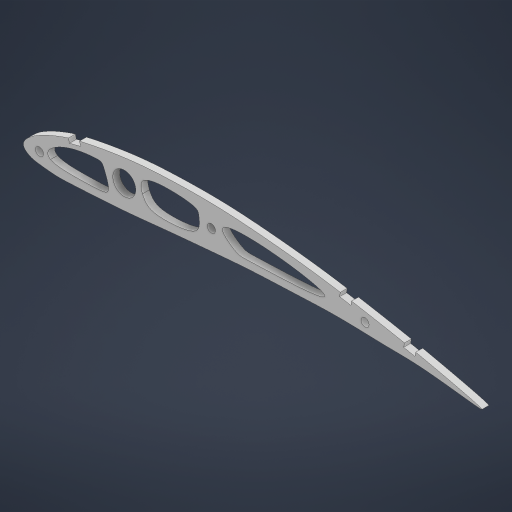
# Autodesk Inventor part: Żebro default
Saved by Autodesk Inventor 2023.2 (Build 272271000, 271)
## iProperties
Created: 2022-12-26
Part Number: Żebro default
Material: Generic
Document SubType Name: Modeling
Designer: Maciej
Density: 1 g/cm^3
Appearance: Default
Author: Maciej
Autodesk Inventor part; units mm, degrees
ref_plane "YZ Plane" through (0, 0, 0) normal (1, 0, 0) x (0, 1, 0)
ref_plane "XZ Plane" through (0, 0, 0) normal (0, 1, 0) x (-1, 0, 0)
ref_plane "XY Plane" through (0, 0, 0) normal (0, 0, 1) x (1, 0, 0)
sketch "Sketch1" plane through (0, 0, 0) normal (0, 0, 1) x (1, 0, 0)
  circle A0 centre (44, 7) radius 5
  spline S0 degree 5 poles (199.9996, -0.38) (200.0106, -0.3312) (199.8804, -0.2049) (199.2285, 0.0711) (197.4897, 0.603) (194.1404, 1.4843) (189.9902, 2.5038) (185.4529, 3.5751) (180.917, 4.6174) (176.6859, 5.5683) (172.905, 6.399) (169.5797, 7.1105) (166.6212, 7.7241) (163.8815, 8.2732) (161.1948, 8.7949) (158.4128, 9.3222) (155.4505, 9.8742) (152.2916, 10.4547) (148.9653, 11.0574) (145.5311, 11.6693) (142.0603, 12.2741) (138.6195, 12.856) (135.2509, 13.4043) (131.9642, 13.9143) (128.7482, 14.3862) (125.5772, 14.8234) (122.4201, 15.231) (119.2476, 15.6147) (116.0409, 15.9792) (112.7977, 16.3273) (109.526, 16.6598) (106.2399, 16.9761) (102.9553, 17.2744) (99.6851, 17.5515) (96.4347, 17.8034) (93.1983, 18.0254) (89.9631, 18.2128) (86.7143, 18.361) (83.4389, 18.467) (80.1306, 18.5292) (76.7936, 18.5484) (73.4478, 18.5285) (70.121, 18.4747) (66.842, 18.3921) (63.6325, 18.2845) (60.4998, 18.1522) (57.4298, 17.991) (54.3776, 17.7904) (51.2803, 17.5356) (48.0737, 17.2117) (44.708, 16.8059) (41.1643, 16.3117) (37.4684, 15.7314) (33.7125, 15.0801) (30.0381, 14.3833) (26.6017, 13.6712) (23.5476, 12.9739) (20.9752, 12.316) (18.9135, 11.7124) (17.2802, 11.1621) (15.8986, 10.6463) (14.5706, 10.1314) (13.1408, 9.567) (11.5443, 8.8974) (9.8001, 8.0944) (8.0206, 7.1907) (6.4035, 6.3015) (5.1063, 5.5301) (4.1412, 4.8917) (3.2339, 4.2107) (2.0734, 3.2532) (0.7635, 1.9494) (-0.1408, 0.4578) (-0.11, -0.9841) (0.869, -2.1755) (2.225, -3.0309) (3.3947, -3.5548) (4.3703, -3.8516) (5.5295, -4.0649) (7.0665, -4.2813) (8.8743, -4.5078) (10.739, -4.7168) (12.4766, -4.8786) (14.0301, -4.9827) (15.4348, -5.0277) (16.824, -5.0185) (18.3985, -4.9615) (20.3559, -4.8641) (22.8188, -4.7325) (25.7852, -4.5706) (29.1702, -4.381) (32.834, -4.1653) (36.6154, -3.9248) (40.3617, -3.661) (43.9625, -3.3764) (47.3772, -3.075) (50.6165, -2.7615) (53.7267, -2.4408) (56.7726, -2.1177) (59.8215, -1.7961) (62.9264, -1.4784) (66.1089, -1.1652) (69.3663, -0.8558) (72.679, -0.5487) (76.0189, -0.2431) (79.3565, 0.0615) (82.6686, 0.3634) (85.9473, 0.6587) (89.1972, 0.9419) (92.4304, 1.2068) (95.6623, 1.4479) (98.9069, 1.6618) (102.1727, 1.8475) (105.4574, 2.0086) (108.7492, 2.1521) (112.0324, 2.2861) (115.292, 2.4185) (118.5181, 2.5543) (121.7099, 2.6948) (124.8823, 2.8347) (128.0632, 2.9627) (131.2839, 3.0653) (134.5721, 3.1297) (137.9424, 3.1463) (141.3901, 3.1121) (144.8796, 3.0338) (148.3468, 2.9283) (151.7203, 2.8162) (154.9369, 2.7175) (157.9613, 2.6462) (160.8018, 2.6058) (163.5319, 2.5834) (166.2946, 2.5476) (169.2559, 2.4601) (172.5682, 2.2839) (176.329, 1.9925) (180.5433, 1.5794) (185.08, 1.0675) (189.6443, 0.5164) (193.8498, 0.0059) (197.2799, -0.3763) (199.0986, -0.515) (199.8149, -0.4977) (199.9887, -0.4288) (199.9996, -0.38) knots 0 0 0 0 0 0 0.007143 0.014286 0.021429 0.028571 0.035714 0.042857 0.05 0.057143 0.064286 0.071429 0.078571 0.085714 0.092857 0.1 0.107143 0.114286 0.121429 0.128571 0.135714 0.142857 0.15 0.157143 0.164286 0.171429 0.178571 0.185714 0.192857 0.2 0.207143 0.214286 0.221429 0.228571 0.235714 0.242857 0.25 0.257143 0.264286 0.271429 0.278571 0.285714 0.292857 0.3 0.307143 0.314286 0.321429 0.328571 0.335714 0.342857 0.35 0.357143 0.364286 0.371429 0.378571 0.385714 0.392857 0.4 0.407143 0.414286 0.421429 0.428571 0.435714 0.442857 0.45 0.457143 0.464286 0.471429 0.478571 0.485714 0.492857 0.5 0.507143 0.514286 0.521429 0.528571 0.535714 0.542857 0.55 0.557143 0.564286 0.571429 0.578571 0.585714 0.592857 0.6 0.607143 0.614286 0.621429 0.628571 0.635714 0.642857 0.65 0.657143 0.664286 0.671429 0.678571 0.685714 0.692857 0.7 0.707143 0.714286 0.721429 0.728571 0.735714 0.742857 0.75 0.757143 0.764286 0.771429 0.778571 0.785714 0.792857 0.8 0.807143 0.814286 0.821429 0.828571 0.835714 0.842857 0.85 0.857143 0.864286 0.871429 0.878571 0.885714 0.892857 0.9 0.907143 0.914286 0.921429 0.928571 0.935714 0.942857 0.95 0.957143 0.964286 0.971429 0.978571 0.985714 0.992857 1 1 1 1 1 1 weights 1 1 1 1 1 1 1 1 1 1 1 1 1 1 1 1 1 1 1 1 1 1 1 1 1 1 1 1 1 1 1 1 1 1 1 1 1 1 1 1 1 1 1 1 1 1 1 1 1 1 1 1 1 1 1 1 1 1 1 1 1 1 1 1 1 1 1 1 1 1 1 1 1 1 1 1 1 1 1 1 1 1 1 1 1 1 1 1 1 1 1 1 1 1 1 1 1 1 1 1 1 1 1 1 1 1 1 1 1 1 1 1 1 1 1 1 1 1 1 1 1 1 1 1 1 1 1 1 1 1 1 1 1 1 1 1 1 1 1 1 1 1 1 1 1
  line L0 (199.9996, -0.38) -> (0, 0) construction
  circle A1 centre (7, 0.4867) radius 1.75
  circle A2 centre (82, 9) radius 1.75
  arc A3 (144.6414, 11.8221) -> (143.8358, 3.0528) centre (149, 7) ccw
  arc A4 (153.9193, 2.7514) -> (154.7671, 9.9984) centre (149, 7) ccw
  circle A5 centre (149, 7) radius 1.75
  spline S1 degree 5 poles (11.8913, -0.0226) (9.7564, 1.1276) (9.8548, 4.1795) (20.0591, 10.8142) (36.7087, 9.5707) (32.968, 11.7598) (40.9835, -3.3233) (34.1297, -0.28) (19.8915, -1.7635) (13.8796, -1.0939) (11.8913, -0.0226) knots 0 0 0 0 0 0 0.226782 0.367091 0.507399 0.673813 0.788783 1 1 1 1 1 1
  line L1 (37.7839, 0.9979) -> (35.0311, -1.1363) construction
  arc A6 (35.282, -0.4902) -> (37.0957, 0.916) centre (35.168, 1.5296) ccw construction
  spline S2 degree 5 poles (51.9512, 7) (51.2364, 8.7392) (50.5608, 11.8889) (51.7504, 15.9179) (81.0563, 13.995) (74.178, 12.4309) (79.8568, 4.5474) (68.6013, 1.7134) (55.8836, 1.6027) (53.8792, 3.3956) (52.5661, 5.5041) (51.9512, 7) knots 0 0 0 0 0 0 0.204171 0.329685 0.4552 0.602697 0.723577 0.824388 1 1 1 1 1 1
  line L2 (77.1203, 5.8641) -> (72.1684, 2.768) construction
  arc A7 (72.5776, 3.4786) -> (76.3022, 5.8074) centre (71.2262, 9.783) ccw construction
  spline S3 degree 5 poles (88.87, 12.7923) (85.9637, 11.8523) (85.6787, 9.3761) (96.1829, 3.8793) (89.8787, 5.0356) (120.8137, 5.278) (153.4075, 7.4889) (108.9137, 14.3324) (93.075, 14.1524) (88.87, 12.7923) knots 0 0 0 0 0 0 0.203943 0.328809 0.528809 0.704922 1 1 1 1 1 1
  line L3 (84.95, 41.5489) -> (116.95, 41.5489)
  line L4 (116.95, 41.5489) -> (116.95, 30.0489)
  line L5 (116.95, 30.0489) -> (84.95, 30.0489)
  line L6 (84.95, 30.0489) -> (84.95, 41.5489)
  circle A8 centre (86.95, 35.7989) radius 1.25
  circle A9 centre (114.95, 35.7989) radius 1.25
  circle A10 centre (106.45, 35.7989) radius 2.5
  line L7 (116.95, 41.5489) -> (112.25, 41.5489)
  line L8 (112.25, 41.5489) -> (112.25, 30.0489)
  line L9 (112.25, 30.0489) -> (116.95, 30.0489)
  line L10 (116.95, 30.0489) -> (116.95, 41.5489)
  line L11 (84.95, 41.5489) -> (89.65, 41.5489)
  line L12 (89.65, 41.5489) -> (89.65, 30.0489)
  line L13 (89.65, 30.0489) -> (84.95, 30.0489)
  line L14 (84.95, 30.0489) -> (84.95, 41.5489)
  line L15 (166.2059, 7.8036) -> (165.8379, 5.9906)
  line L16 (165.8379, 5.9906) -> (170.738, 4.9959)
  line L17 (170.738, 4.9959) -> (171.1191, 6.7785)
  line L18 (126.7322, 6.3766) -> (131.9817, 7.6234) construction
  arc A11 (127.2429, 6.6476) -> (131.4037, 7.6358) centre (125.7133, 22.3417) ccw construction
  line L19 (24.478, 13.1758) -> (24.9322, 11.434)
  line L20 (24.9322, 11.434) -> (20.094, 10.1724)
  line L21 (20.094, 10.1724) -> (19.6398, 11.9142)
  line L22 (138.2023, 12.9196) -> (137.9018, 11.1449)
  line L23 (137.9018, 11.1449) -> (142.8317, 10.3102)
  line L24 (142.8317, 10.3102) -> (143.1322, 12.0849)
  point P0 (33.7236, 10.1341)
  point P1 (35.6581, 7)
  point P2 (36.4075, -0.0692)
  point P3 (75.8381, 12.7923)
  point P4 (76.6928, 9.6078)
  point P5 (74.6444, 4.316)
  point P6 (55.9638, 2.7971)
  point P7 (94.2398, 4.9953)
  point P8 (129.3569, 7)
  point P9 (84.95, 35.7989)
  point P10 (116.95, 35.7989)
  point P11 (183.35, 1.2569)
  point P12 (188.3021, 0.6772)
  dimension "d0" = 200
  dimension "d1" = 3.5
  dimension "d5" = 2
  dimension "d12" = 44
  dimension "d13" = 7
  dimension "d14" = 10
  dimension "d15" = 37
  dimension "d18" = 38
  dimension "d20" = 6.5
  dimension "d21" = 6.5
  dimension "d23" = 3.5
  dimension "d24" = 105
  dimension "d25" = 0.5
  dimension "d26" = 3.5
  dimension "d27" = 32
  dimension "d28" = 11.5
  dimension "d29" = 2.5
  dimension "d30" = 2.5
  dimension "d31" = 2
  dimension "d32" = 2
  dimension "d34" = 10.5
  dimension "d35" = 5
  dimension "d36" = 4.7
  dimension "d37" = 4.7
  dimension "d39" = 1.85
  dimension "d40" = 5
  dimension "d41" = 1.8229
  dimension "d49" = 5
  dimension "d50" = 1.8
  dimension "d51" = 5
  dimension "d52" = 1.8
  constraints: 50 end point, 12 centre point, 8 midpoint, 8 parallel, 7 point on circle, 4 horizontal alignment, 4 perpendicular, 4 point on line, 3 horizontal, 2 coincident, 49 other
  measures "d0" distance of L0.start L0.end
  measures "d1" diameter of A1
  measures "d5" vertical distance of A0.centre A2.centre
  measures "d12" horizontal distance of L0.end A0.centre
  measures "d13" vertical distance of L0.end A0.centre
  measures "d14" diameter of A0
  measures "d15" horizontal distance of A0.centre A1.centre
  measures "d18" horizontal distance of A0.centre A2.centre
  measures "d20" radius of A4
  measures "d21" radius of A3
  measures "d23" diameter of A5
  measures "d24" distance of A0.centre A3.centre
  measures "d25" distance from line of L0 A1.centre
  measures "d26" diameter of A2
  measures "d27" distance of L4.end L5.end
  measures "d28" distance of L3.end L4.end
  measures "d29" diameter of A8
  measures "d30" diameter of A9
  measures "d31" distance from line of L6 A8.centre
  measures "d32" distance from line of L4 A9.centre
  measures "d34" distance from line of L4 A10.centre
  measures "d35" diameter of A10
  measures "d36" distance of L9.end L8.end
  measures "d37" distance of L12.end L13.end
  measures "d39" distance of L15.start L15.end
  measures "d40" distance of L15.end L16.end
  measures "d41" distance of L16.end L17.end
  measures "d49" distance of L21.end L19.start
  measures "d50" distance of L19.start L19.end
  measures "d51" distance of L24.end L22.start
  measures "d52" distance of L22.end L22.start
extrude "Extrusion1" add sketch "Sketch1" along normal blind 3 contours S0 A4 L15 L16 L17 | S0 A3 A4 | S0 L21 L20 L19 L22 L23 L24 A3
body "Solid1"
